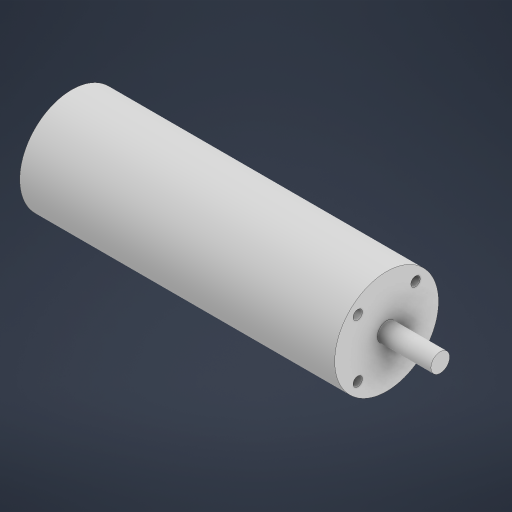
# Autodesk Inventor part: MOOOOT
Saved by Autodesk Inventor 2023 (Build 270158000, 158)
## iProperties
Created: 2023-09-11
Part Number: MOOOOT
Material: Generic
Document SubType Name: Modeling
Designer: Abhinav
Density: 1 g/cm^3
Appearance: Default
Author: Abhinav
Autodesk Inventor part; units mm, degrees
ref_plane "YZ Plane" through (0, 0, 0) normal (1, 0, 0) x (0, 1, 0)
ref_plane "XZ Plane" through (0, 0, 0) normal (0, 1, 0) x (-1, 0, 0)
ref_plane "XY Plane" through (0, 0, 0) normal (0, 0, 1) x (1, 0, 0)
sketch "Sketch1" plane through (0, 0, 0) normal (1, 0, 0) x (0, 1, 0)
  circle A0 centre (0, 0) radius 22.25
  dimension "d0" = 44.5
  constraints: 1 centre point, 1 coincident
  measures "d0" diameter of A0
extrude "Extrusion1" add sketch "Sketch1" along normal blind 135
sketch "Sketch2" plane through (135, 0, 0) normal (1, 0, 0) x (0, 0, -1)
  circle A0 centre (0, 0) radius 4
  line L0 (0, 0) -> (12.3744, 12.3744) construction
  line L1 (0, 0) -> (17.5, 0) construction
  line L2 (0, 0) -> (-12.3744, -12.3744) construction
  line L3 (0, 0) -> (17.5, 0) construction
  circle A1 centre (-12.3744, -12.3744) radius 2
  circle A2 centre (12.3744, 12.3744) radius 2
  circle A3 centre (-12.3744, 12.3744) radius 2
  circle A4 centre (12.3744, -12.3744) radius 2
  circle A5 centre (0, 0) radius 17.5 construction
  dimension "d3" = 8
  dimension "d6" = 17.5
  dimension "d7" = 45
  dimension "d8" = 17.5
  dimension "d9" = 135
  dimension "d10" = 4
  dimension "d11" = 4
  constraints: 8 end point, 5 centre point, 4 coincident, 2 equal length, 2 horizontal, 2 symmetric about line, 5 other
  measures "d3" diameter of A0
  measures "d6" distance of L0.start L0.end
  measures "d7" angle of L1 L0
  measures "d8" distance of L0.start L2.end
  measures "d9" angle of L2 L3
  measures "d10" diameter of A1
  measures "d11" diameter of A2
extrude "Extrusion2" add sketch "Sketch2" along normal blind 23 contours A0
extrude "Extrusion3" cut sketch "Sketch2" against normal blind 5 contours A1 | A2 | A3 | A4
body "Solid1"
